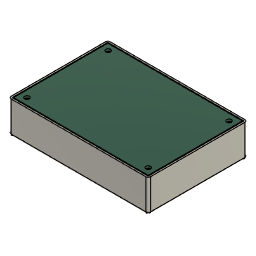
Commodore_KB_Tester_Rev2 v2 (Autodesk Fusion 360 design; units mm, degrees)
Autodesk Fusion 360 part; units mm, degrees
sketch "Sketch1" plane through (0, 0, 0) normal (0, 0, 1) x (1, 0, 0) in component "PCB"
  line L0 (100, 0) -> (100, 70)
  circle A0 centre (52, 35) radius 3.1
  circle A1 centre (35, 27) radius 3.1
  circle A2 centre (35, 42) radius 3.1
  line L1 (0, 0) -> (100, 0)
  line L2 (0, 70) -> (0, 0)
  circle A3 centre (52, 41.4) radius 1.2
  circle A4 centre (28.6, 27) radius 1.2
  line L3 (100, 70) -> (0, 70)
  circle A5 centre (28.6, 42) radius 1.2
  line L4 (99.15, 22.18) -> (97.6, 22.18)
  line L5 (97.6, 22.18) -> (97.6, 15.02)
  line L6 (88.4, 15.02) -> (97.6, 15.02)
  line L7 (97.6, 15.02) -> (99.15, 15.02)
  line L8 (97.6, 22.18) -> (88.4, 22.18)
  line L9 (94.5, 22.84) -> (94.7, 22.64)
  line L10 (94.7, 22.64) -> (93.4, 22.64)
  line L11 (93.4, 22.84) -> (93.4, 22.44)
  line L12 (99.15, 15.02) -> (99.15, 22.18)
  line L13 (72.2313, 9.5251) -> (67.6275, 9.5251)
  line L14 (72.2313, 8.5725) -> (72.2313, 9.5251)
  circle A6 centre (5, 5) radius 3.1789
  line L15 (2.54, 60) -> (2.54, 59)
  line L16 (2.54, 49.4) -> (2.54, 47.2)
  line L17 (14.04, 42) -> (18.34, 42)
  arc A7 (18.34, 49) -> (19.04, 49.7) centre (18.34, 49.7) ccw
  line L18 (18.34, 45.5) -> (16.54, 45.5)
  line L19 (67.6276, 8.5725) -> (72.2313, 8.5725)
  arc A8 (19.04, 52.3) -> (18.34, 53) centre (18.34, 52.3) ccw
  line L20 (2.54, 52.6) -> (2.54, 49.4)
  circle A9 centre (95, 65) radius 1.7463
  line L21 (2.54, 54.8) -> (2.54, 52.6)
  circle A10 centre (5, 5) radius 1.7463
  line L22 (19.04, 49.7) -> (19.04, 52.3)
  arc A11 (18.34, 42) -> (19.04, 42.7) centre (18.34, 42.7) ccw
  line L23 (67.6275, 9.5251) -> (67.6276, 8.5725)
  circle A12 centre (95, 65) radius 3.1789
  line L24 (16.54, 33) -> (18.34, 33)
  line L25 (19.04, 42.7) -> (19.04, 44.8)
  line L26 (13.64, 43) -> (14.04, 43)
  line L27 (16.04, 58.1) -> (16.34, 58.1)
  line L28 (2.54, 43) -> (1.54, 43)
  line L29 (2.54, 49.4) -> (14.04, 49.4)
  line L30 (14.04, 49.4) -> (14.04, 46.6)
  arc A13 (19.04, 59.3) -> (18.34, 60) centre (18.34, 59.3) ccw
  line L31 (2.54, 23) -> (2.54, 22)
  arc A14 (19.04, 44.8) -> (18.34, 45.5) centre (18.34, 44.8) ccw
  line L32 (18.34, 25.5) -> (16.54, 25.5)
  line L33 (0.84, 61.6) -> (0.84, 60)
  line L34 (14.04, 59) -> (14.04, 56.6)
  circle A15 centre (95, 5) radius 1.7463
  line L35 (0.74, 40.4) -> (0.74, 42)
  arc A16 (18.34, 22) -> (19.04, 22.7) centre (18.34, 22.7) ccw
  line L36 (1.54, 43) -> (1.54, 40.4)
  line L37 (18.34, 56.5) -> (16.54, 56.5)
  line L38 (2.54, 43) -> (11.44, 43)
  line L39 (0.04, 61.6) -> (0.04, 42)
  line L40 (2.54, 44.8) -> (2.54, 43)
  line L41 (1.54, 59) -> (2.54, 59)
  arc A17 (19.04, 24.8) -> (18.34, 25.5) centre (18.34, 24.8) ccw
  line L42 (16.34, 58.9) -> (16.04, 58.9)
  line L43 (2.54, 52.6) -> (14.04, 52.6)
  line L44 (14.04, 55.4) -> (14.04, 52.6)
  line L45 (14.04, 45.4) -> (14.04, 43)
  line L46 (16.04, 58.9) -> (16.04, 58.1)
  line L47 (2.54, 42) -> (14.04, 42)
  line L48 (16.54, 53) -> (18.34, 53)
  line L49 (2.54, 40) -> (2.54, 39)
  line L50 (2.54, 32.6) -> (2.54, 29.4)
  circle A18 centre (4.99, 65.33) radius 1.7463
  line L51 (2.54, 29.4) -> (2.54, 27.2)
  line L52 (16.54, 56.5) -> (16.54, 53)
  line L53 (2.54, 39) -> (2.54, 37.2)
  line L54 (16.54, 49) -> (18.34, 49)
  arc A19 (19.04, 32.3) -> (18.34, 33) centre (18.34, 32.3) ccw
  line L55 (0.74, 42) -> (0.04, 42)
  line L56 (2.54, 59) -> (2.54, 57.2)
  line L57 (14.04, 43) -> (14.04, 42)
  line L58 (0.84, 60) -> (1.54, 60)
  line L59 (16.04, 43.9) -> (16.04, 43.1)
  line L60 (2.54, 24.8) -> (2.54, 23)
  line L61 (16.34, 43.9) -> (16.04, 43.9)
  line L62 (2.54, 43) -> (2.54, 42)
  line L63 (14.04, 60) -> (2.54, 60)
  line L64 (14.04, 52.6) -> (14.04, 49.4)
  line L65 (16.54, 49) -> (16.54, 45.5)
  line L66 (0.74, 40.4) -> (1.54, 40.4)
  circle A20 centre (4.99, 65.33) radius 3.1789
  line L67 (2.54, 34.8) -> (2.54, 32.6)
  line L68 (16.04, 43.1) -> (16.34, 43.1)
  circle A21 centre (95, 5) radius 3.1789
  line L69 (1.54, 60) -> (1.54, 59)
  arc A22 (18.34, 56.5) -> (19.04, 57.2) centre (18.34, 57.2) ccw
  line L70 (0.04, 61.6) -> (0.84, 61.6)
  line L71 (13.64, 59) -> (14.04, 59)
  line L72 (14.04, 40) -> (14.04, 39)
  arc A23 (19.04, 39.3) -> (18.34, 40) centre (18.34, 39.3) ccw
  line L73 (18.34, 60) -> (14.04, 60)
  line L74 (16.04, 23.9) -> (16.04, 23.1)
  line L75 (14.5, 16.5) -> (14, 16.5)
  line L76 (19.04, 22.7) -> (19.04, 24.8)
  line L77 (14.04, 35.4) -> (14.04, 32.6)
  line L78 (14.04, 22) -> (18.34, 22)
  line L79 (18.34, 40) -> (14.04, 40)
  line L80 (16.04, 38.9) -> (16.04, 38.1)
  line L81 (16.04, 23.1) -> (18.04, 23.1)
  line L82 (2.54, 23) -> (1.54, 23)
  line L83 (2.54, 29.4) -> (14.04, 29.4)
  line L84 (0.04, 41.6) -> (0.84, 41.6)
  line L85 (14, 19.5) -> (14, 19.2)
  line L86 (3.5, 19.2) -> (3.5, 19.5)
  line L87 (18.34, 36.5) -> (16.54, 36.5)
  line L88 (14.04, 40) -> (2.54, 40)
  line L89 (14.04, 29.4) -> (14.04, 26.6)
  line L90 (0.74, 20.4) -> (0.74, 22)
  line L91 (14.04, 39) -> (14.04, 36.6)
  line L92 (0.74, 22) -> (0.04, 22)
  line L93 (16.54, 29) -> (18.34, 29)
  line L94 (14.04, 32.6) -> (14.04, 29.4)
  line L95 (19.04, 29.7) -> (19.04, 32.3)
  line L96 (1.54, 39) -> (2.54, 39)
  line L97 (13.64, 23) -> (14.04, 23)
  line L98 (16.54, 29) -> (16.54, 25.5)
  line L99 (14.5, 16.5) -> (14.5, 19.5)
  line L100 (16.54, 36.5) -> (16.54, 33)
  line L101 (18.04, 23.9) -> (16.04, 23.9)
  line L102 (1.54, 23) -> (1.54, 20.4)
  line L103 (0.84, 40) -> (1.54, 40)
  line L104 (18.04, 38.9) -> (16.04, 38.9)
  line L105 (2.54, 23) -> (11.44, 23)
  line L106 (1.54, 40) -> (1.54, 39)
  line L107 (16.04, 38.1) -> (18.04, 38.1)
  line L108 (91.3, 57.912) -> (91.4232, 57.912)
  line L109 (0.74, 20.4) -> (1.54, 20.4)
  line L110 (18.04, 38.1) -> (18.04, 38.9)
  line L111 (18.04, 23.1) -> (18.04, 23.9)
  line L112 (14.5, 13.5) -> (14.5, 13.8)
  line L113 (14, 19.2) -> (14, 16.5)
  line L114 (11.5, 10.8) -> (14, 10.8)
  line L115 (91.3, 58) -> (91.3, 57)
  line L116 (2.54, 59) -> (11.44, 59)
  line L117 (13.64, 39) -> (14.04, 39)
  line L118 (3.5, 10.8) -> (9.7, 10.8)
  arc A24 (18.34, 29) -> (19.04, 29.7) centre (18.34, 29.7) ccw
  line L119 (14.04, 23) -> (14.04, 22)
  arc A25 (18.34, 36.5) -> (19.04, 37.2) centre (18.34, 37.2) ccw
  line L120 (0.84, 41.6) -> (0.84, 40)
  line L121 (19.04, 39.3) -> (19.04, 37.2)
  line L122 (2.54, 22) -> (14.04, 22)
  line L123 (0.04, 41.6) -> (0.04, 22)
  line L124 (2.54, 32.6) -> (14.04, 32.6)
  line L125 (99.15, 43.96) -> (99.15, 59.04)
  line L126 (14.04, 60) -> (14.04, 59)
  line L127 (97.6, 59.04) -> (88.4, 59.04)
  line L128 (14.04, 25.4) -> (14.04, 23)
  line L129 (2.54, 39) -> (11.44, 39)
  line L130 (91.3, 21.14) -> (91.3, 20.14)
  line L131 (3.5, 10.8) -> (3.5, 19.2)
  line L132 (88.4, 22.18) -> (88.4, 15.02)
  line L133 (14.5, 10.5) -> (14, 10.5)
  line L134 (97.6, 29.44) -> (99.15, 29.44)
  line L135 (91.3, 57.15) -> (91.51, 57.15)
  line L136 (91.3, 57.785) -> (91.601, 57.785)
  line L137 (91.3, 57.531) -> (91.9566, 57.531)
  line L138 (97.6, 40.56) -> (88.4, 40.56)
  line L139 (97.6, 59.04) -> (97.6, 43.96)
  line L140 (92, 57.5) -> (91.3, 58)
  line L141 (91.3, 57.658) -> (91.7788, 57.658)
  line L142 (91.3, 39.37) -> (91.51, 39.37)
  line L143 (88.4, 29.44) -> (97.6, 29.44)
  line L144 (14, 13.5) -> (14, 10.8)
  line L145 (92, 39.02) -> (91.3, 39.52)
  line L146 (91.3, 39.243) -> (91.6878, 39.243)
  line L147 (3.5, 10.5) -> (3.5, 10.8)
  line L148 (99.15, 29.44) -> (99.15, 40.56)
  line L149 (91.3, 39.52) -> (91.3, 38.52)
  line L150 (91.3, 21.082) -> (91.3812, 21.082)
  line L151 (88.4, 59.04) -> (88.4, 43.96)
  line L152 (14, 13.5) -> (14.5, 13.5)
  line L153 (14.5, 13.5) -> (14.5, 10.5)
  line L154 (91.3, 57) -> (92, 57.5)
  line L155 (91.3, 57.023) -> (91.3322, 57.023)
  line L156 (91.3, 20.955) -> (91.559, 20.955)
  line L157 (94.7, 41.02) -> (93.4, 41.02)
  line L158 (14.5, 19.5) -> (14, 19.5)
  line L159 (14, 13.8) -> (14, 13.5)
  line L160 (14, 10.8) -> (14, 10.5)
  line L161 (91.3, 38.52) -> (92, 39.02)
  line L162 (0, 10.5) -> (3.5, 10.5)
  line L163 (94.5, 59.7) -> (94.7, 59.5)
  line L164 (93.4, 59.7) -> (93.4, 59.3)
  line L165 (88.4, 43.96) -> (97.6, 43.96)
  line L166 (97.6, 43.96) -> (99.15, 43.96)
  line L167 (91.3, 57.277) -> (91.6878, 57.277)
  line L168 (91.3, 57.404) -> (91.8656, 57.404)
  line L169 (14, 16.5) -> (14, 16.2)
  line L170 (91.3, 39.116) -> (91.8656, 39.116)
  line L171 (3.5, 19.5) -> (0, 19.5)
  line L172 (91.3, 20.447) -> (91.7298, 20.447)
  line L173 (91.3, 20.574) -> (91.9076, 20.574)
  line L174 (9.5, 10.5) -> (3.5, 10.5)
  line L175 (3.5, 19.5) -> (14, 19.5)
  line L176 (3.5, 19.2) -> (14, 19.2)
  line L177 (91.3, 20.193) -> (91.3742, 20.193)
  line L178 (14.5, 16.5) -> (14.5, 16.2)
  line L179 (91.3, 20.32) -> (91.552, 20.32)
  line L180 (91.3, 20.701) -> (91.9146, 20.701)
  line L181 (0, 19.5) -> (0, 10.5)
  line L182 (91.3, 20.828) -> (91.7368, 20.828)
  line L183 (91.3, 39.497) -> (91.3322, 39.497)
  line L184 (99.15, 59.04) -> (97.6, 59.04)
  line L185 (88.4, 40.56) -> (88.4, 29.44)
  line L186 (91.3, 20.14) -> (92, 20.64)
  line L187 (99.15, 40.56) -> (97.6, 40.56)
  line L188 (14, 10.5) -> (11.7, 10.5)
  line L189 (94.7, 59.5) -> (93.4, 59.5)
  line L190 (91.3, 38.862) -> (91.7788, 38.862)
  line L191 (91.3, 38.989) -> (91.9566, 38.989)
  line L192 (94.5, 41.22) -> (94.7, 41.02)
  arc A26 (38.7, 28.1) -> (38.7, 25.85) centre (34.9998, 26.975) ccw
  line L193 (37.25, 30.85) -> (32.75, 30.85)
  line L194 (92, 20.64) -> (91.3, 21.14)
  circle A27 centre (52, 35) radius 5.4
  line L195 (37.25, 30.85) -> (39.45, 27)
  circle A28 centre (35, 42) radius 5.4
  arc A29 (37.7, 25.5) -> (37.7, 28.5) centre (37.7, 27) ccw
  line L196 (39.45, 27) -> (37.25, 23.15)
  line L197 (93.4, 41.22) -> (93.4, 40.82)
  line L198 (91.3, 38.735) -> (91.601, 38.735)
  line L199 (91.3, 38.608) -> (91.4232, 38.608)
  line L200 (37.25, 45.85) -> (39.45, 42)
  line L201 (30.55, 42) -> (32.75, 38.15)
  line L202 (32.75, 45.85) -> (30.55, 42)
  line L203 (32.75, 30.85) -> (30.55, 27)
  line L204 (39.45, 42) -> (37.25, 38.15)
  line L205 (37.25, 23.15) -> (32.75, 23.15)
  circle A30 centre (35, 27) radius 5.4
  line L206 (55.85, 32.75) -> (52, 30.55)
  line L207 (52, 30.55) -> (48.15, 32.75)
  line L208 (30.55, 27) -> (32.75, 23.15)
  line L209 (37.25, 38.15) -> (32.75, 38.15)
  line L210 (55.85, 32.75) -> (55.85, 37.25)
  arc A31 (53.1, 31.3) -> (50.85, 31.3) centre (51.975, 35.0002) ccw
  arc A32 (38.7, 43.1) -> (38.7, 40.85) centre (34.9998, 41.975) ccw
  line L211 (37.25, 45.85) -> (32.75, 45.85)
  line L212 (48.15, 32.75) -> (48.15, 37.25)
  line L213 (52, 39.45) -> (48.15, 37.25)
  line L214 (55.85, 37.25) -> (52, 39.45)
  line L215 (97.6, 40.56) -> (97.6, 29.44)
  arc A33 (37.7, 40.5) -> (37.7, 43.5) centre (37.7, 42) ccw
  arc A34 (50.5, 32.3) -> (53.5, 32.3) centre (52, 32.3) ccw
  line L216 (93.4, 21.18) -> (93.4, 19.98)
  line L217 (94.6, 17.22) -> (93.4, 17.22)
  line L218 (93.4, 16.02) -> (94.6, 16.02)
  line L219 (93.4, 19.98) -> (94.6, 19.98)
  line L220 (94.6, 21.18) -> (93.4, 21.18)
  line L221 (93.4, 17.22) -> (93.4, 16.02)
  line L222 (18.04, 58.1) -> (18.04, 58.9)
  circle A35 centre (43, 9) radius 2
  line L223 (2.54, 57.2) -> (2.54, 54.8)
  circle A36 centre (62.05, 9) radius 5
  circle A37 centre (43, 61) radius 5
  line L224 (2.54, 37.2) -> (2.54, 34.8)
  line L225 (18.04, 58.9) -> (16.34, 58.9)
  circle A38 centre (62.05, 9) radius 2
  line L226 (93.4, 58.04) -> (93.4, 56.84)
  line L227 (14.04, 46.6) -> (14.04, 45.4)
  line L228 (94.6, 16.02) -> (94.6, 17.22)
  line L229 (18.04, 43.1) -> (18.04, 43.9)
  line L230 (16.34, 43.1) -> (18.04, 43.1)
  line L231 (94.6, 19.98) -> (94.6, 21.18)
  line L232 (11.44, 43) -> (13.64, 43)
  line L233 (14.04, 56.6) -> (14.04, 55.4)
  circle A39 centre (43, 9) radius 5
  line L234 (2.54, 47.2) -> (2.54, 44.8)
  circle A40 centre (78, 61) radius 2
  line L235 (14.04, 26.6) -> (14.04, 25.4)
  circle A41 centre (78, 9) radius 2
  line L236 (2.54, 27.2) -> (2.54, 24.8)
  circle A42 centre (78, 61) radius 5
  circle A43 centre (62.05, 61) radius 2
  circle A44 centre (78, 41.95) radius 2
  circle A45 centre (78, 28.05) radius 2
  circle A46 centre (78, 41.95) radius 5
  line L237 (11.44, 23) -> (13.64, 23)
  circle A47 centre (62.05, 61) radius 5
  line L238 (14.04, 36.6) -> (14.04, 35.4)
  line L239 (14, 16.2) -> (14, 13.8)
  line L240 (18.04, 43.9) -> (16.34, 43.9)
  line L241 (11.44, 39) -> (13.64, 39)
  circle A48 centre (43, 61) radius 2
  line L242 (16.34, 58.1) -> (18.04, 58.1)
  line L243 (10, 10.5) -> (11.2, 10.5)
  line L244 (11.44, 59) -> (13.64, 59)
  line L245 (11.2, 10) -> (10, 10)
  circle A49 centre (78, 9) radius 5
  line L246 (93.4, 56.84) -> (94.6, 56.84)
  line L247 (14.5, 13.8) -> (14.5, 16.2)
  line L248 (94.6, 35.6) -> (93.4, 35.6)
  line L249 (36.45, 28.5) -> (37.5, 28.5)
  line L250 (94.6, 31.64) -> (93.4, 31.64)
  line L251 (36.45, 43.5) -> (37.5, 43.5)
  line L252 (53.5, 35) -> (53.5, 33.55)
  line L253 (94.6, 46.16) -> (93.4, 46.16)
  line L254 (94.6, 39.56) -> (93.4, 39.56)
  line L255 (94.6, 56.84) -> (94.6, 58.04)
  line L256 (93.4, 52.88) -> (94.6, 52.88)
  line L257 (10, 10) -> (10, 10.5)
  line L258 (9.7, 10.8) -> (11.5, 10.8)
  line L259 (94.6, 38.36) -> (94.6, 39.56)
  line L260 (93.4, 48.92) -> (94.6, 48.92)
  line L261 (94.6, 48.92) -> (94.6, 50.12)
  arc A50 (53.5, 32.5) -> (50.5, 32.5) centre (52, 35) ccw
  line L262 (36.45, 40.5) -> (37.5, 40.5)
  line L263 (94.6, 54.08) -> (93.4, 54.08)
  arc A51 (36.45, 43.5) -> (36.45, 40.5) centre (35, 42) ccw
  arc A52 (37.5, 43.5) -> (37.5, 40.5) centre (35, 42) ccw
  line L264 (37.5, 28.5) -> (37.7, 28.5)
  line L265 (93.4, 31.64) -> (93.4, 30.44)
  line L266 (35, 25.5) -> (36.45, 25.5)
  line L267 (94.6, 34.4) -> (94.6, 35.6)
  line L268 (93.4, 46.16) -> (93.4, 44.96)
  line L269 (94.6, 44.96) -> (94.6, 46.16)
  line L270 (93.4, 30.44) -> (94.6, 30.44)
  line L271 (93.4, 50.12) -> (93.4, 48.92)
  line L272 (11.2, 10.5) -> (11.7, 10.5)
  line L273 (93.4, 34.4) -> (94.6, 34.4)
  line L274 (93.4, 35.6) -> (93.4, 34.4)
  line L275 (50.5, 35) -> (50.5, 33.55)
  line L276 (94.6, 52.88) -> (94.6, 54.08)
  line L277 (50.5, 32.5) -> (50.5, 32.3)
  line L278 (36.45, 25.5) -> (37.5, 25.5)
  line L279 (37.5, 25.5) -> (37.7, 25.5)
  line L280 (35, 28.5) -> (36.45, 28.5)
  circle A53 centre (78, 28.05) radius 5
  line L281 (9.5, 10.5) -> (10, 10.5)
  line L282 (11.2, 10.5) -> (11.2, 10)
  line L283 (37.5, 40.5) -> (37.7, 40.5)
  line L284 (93.4, 54.08) -> (93.4, 52.88)
  line L285 (94.6, 50.12) -> (93.4, 50.12)
  line L286 (53.5, 33.55) -> (53.5, 32.5)
  line L287 (93.4, 44.96) -> (94.6, 44.96)
  line L288 (94.6, 30.44) -> (94.6, 31.64)
  line L289 (94.6, 58.04) -> (93.4, 58.04)
  line L290 (35, 43.5) -> (36.45, 43.5)
  arc A54 (53.5, 35) -> (50.5, 35) centre (52, 35) ccw
  arc A55 (53.5, 33.55) -> (50.5, 33.55) centre (52, 35) ccw
  line L291 (35, 40.5) -> (36.45, 40.5)
  line L292 (93.4, 39.56) -> (93.4, 38.36)
  arc A56 (37.5, 28.5) -> (37.5, 25.5) centre (35, 27) ccw
  line L293 (93.4, 38.36) -> (94.6, 38.36)
  arc A57 (36.45, 28.5) -> (36.45, 25.5) centre (35, 27) ccw
  line L294 (53.5, 32.5) -> (53.5, 32.3)
  arc A58 (35, 28.5) -> (35, 25.5) centre (35, 27) ccw
  arc A59 (35, 43.5) -> (35, 40.5) centre (35, 42) ccw
  line L295 (37.5, 43.5) -> (37.7, 43.5)
  line L296 (50.5, 33.55) -> (50.5, 32.5)
  line L297 (-50, -35) -> (50, -35) construction
  line L298 (50, -35) -> (50, 35) construction
  line L299 (50, 35) -> (-50, 35) construction
  line L300 (-50, 35) -> (-50, -35) construction
  circle A60 centre (-45.01, 30.33) radius 1.7463 construction
  circle A61 centre (45, 30) radius 1.7463 construction
  circle A62 centre (45, -30) radius 1.7463 construction
  circle A63 centre (-45, -30) radius 1.7463 construction
extrude "Extrude1" add sketch "Sketch1" along normal blind 1.6 contours L0 L1 L2 L3 L99 L112 L133 L153 L158 L162 L171 L174 L175 L178 L188 L245 L247 L257 L272 L281 L282 | L2 L86 L131 L147 L162 L171 L181 | L114 L118 L147 L160 L174 L188 L243 L258 L272 L281 | L85 L86 L175 L176 | L113 L114 L118 L131 L144 L159 L169 L176 L239 L258 | L75 L85 L99 L113 L158 | L243 L245 L257 L282 | L75 L112 L152 L159 L169 L178 L239 L247 | L133 L144 L152 L153 L160 | A0 A34 A50 L277 L294 | A0 A34 L252 L275 L277 L286 A54 L294 L296 | A0 A34 | A50 L286 A55 L296 | L252 L275 A54 A55 | A1 A29 L249 L264 L266 L278 L279 L280 A58 | A1 A29 | A1 A29 L264 L279 A56 | L249 L278 A56 A57 | L266 L280 A57 A58 | A2 A33 L251 L262 L283 L290 L291 A59 L295 | A2 A33 | A2 A33 A52 L283 L295 | L251 L262 A51 A52 | A51 L290 L291 A59 | A3 A27 | A3 A27 | A3 A27 | A4 A30 | A4 A30 | A4 A30 | A5 A28 | A5 A28 | A5 A28 | L4 L5 L7 L12 | L5 L6 L8 L132 | L13 L14 L19 L23 | A6 | L15 L63 L71 L116 L126 L244 | L16 L20 L21 L28 L33 L35 L36 L39 L40 L41 L55 L56 L58 L66 L69 L70 L84 L120 L223 L234 | L21 L34 L43 L44 L56 L71 L116 L223 L233 L244 | L20 L29 L43 L64 | L16 L26 L29 L30 L38 L40 L45 L227 L232 L234 | L26 L38 L47 L57 L62 L232 | L35 L66 L84 L120 | L35 L50 L51 L53 L60 L66 L67 L82 L84 L90 L92 L96 L102 L103 L106 L109 L120 L123 L224 L236 | L53 L67 L77 L91 L117 L124 L129 L224 L238 L241 | L49 L72 L88 L117 L129 L241 | L31 L97 L105 L119 L122 L237 | L51 L60 L83 L89 L97 L105 L128 L235 L236 L237 | L24 L32 A16 A17 A19 L72 A23 L76 L77 L78 L79 L87 L89 L91 L93 L94 L95 L98 L100 A24 L119 A25 L121 L128 L235 L238 | L50 L83 L94 L124 | A12 | L27 L42 L46 L222 L225 L242 | L59 L61 L68 L229 L230 L240 | A20 | A21 | L74 L81 L101 L111 | L80 L104 L107 L110 | L108 L115 L140 | L108 L115 L136 L140 | L115 L136 L140 L141 | L115 L137 L140 L141 | L115 L137 L140 L154 L168 | L115 L154 L167 L168 | L115 L135 L154 L167 | L115 L135 L154 L155 | L115 L154 L155 | L125 L139 L166 L184 | L127 L139 L151 L165 | L130 L150 L194 | L130 L150 L156 L194 | L130 L156 L182 L194 | L130 L180 L182 L194 | L130 L173 L180 L186 L194 | L130 L172 L173 L186 | L130 L172 L179 L186 | L130 L177 L179 L186 | L130 L177 L186 | L134 L148 L187 L215 | L138 L143 L185 L215 | L142 L145 L149 L183 | L142 L145 L146 L149 | L145 L149 L183 | L145 L146 L149 L170 | L145 L149 L161 L170 L191 | L149 L161 L190 L191 | L149 L161 L190 L198 | L149 L161 L198 L199 | L149 L161 L199 | A26 L208 | A26 L193 L195 L196 L203 L205 L208 | A26 L205 L208 | A26 L205 | A26 L196 L205 | A26 L196 | L200 L201 L202 L204 L209 A32 L211 | L204 A32 | L204 L209 A32 | L201 A32 | L209 A32 | L201 L209 A32 | L206 L207 L210 A31 L212 L213 L214 | L207 A31 | L207 A31 L212 | A31 L213 | A31 L212 | A31 L212 L213 | L216 L219 L220 L231 | L217 L218 L221 L228 | A35 | A36 | A37 | A38 | L226 L246 L255 L289 | A39 | A40 | A41 | A42 | A43 | A44 | A45 | A46 | A47 | A48 | A49 | L248 L267 L273 L274 | L250 L265 L270 L288 | L253 L268 L269 L287 | L254 L259 L292 L293 | L256 L263 L276 L284 | L260 L261 L271 L285 | A53 makes body 1 in component "PCB"
ref_plane "WorkPlane1" through (50, 35, -21) normal (0, 0, 1) x (1, 0, 0) in component "KB_Tester_bottom_shell_Rev2"
sketch "Sketch1 (2)" plane through (50, 35, -21) normal (0, 0, 1) x (1, 0, 0) in component "KB_Tester_bottom_shell_Rev2"
  line L0 (-50, -35) -> (50, -35) construction
  line L1 (50, -35) -> (50, 35) construction
  line L2 (50, 35) -> (-50, 35) construction
  line L3 (-50, 35) -> (-50, -35) construction
  circle A0 centre (-45.01, 30.33) radius 1.7463 construction
  circle A1 centre (45, 30) radius 1.7463 construction
  circle A2 centre (45, -30) radius 1.7463 construction
  circle A3 centre (-45, -30) radius 1.7463 construction
  line L4 (50, -35.5) -> (-50, -35.5)
  line L5 (-50.5, -35) -> (-50.5, 35)
  line L6 (-50, 35.5) -> (50, 35.5)
  line L7 (50.5, 35) -> (50.5, -35)
  arc A4 (50.5, 35) -> (50, 35.5) centre (50, 35) ccw
  arc A5 (-50, 35.5) -> (-50.5, 35) centre (-50, 35) ccw
  arc A6 (-50.5, -35) -> (-50, -35.5) centre (-50, -35) ccw
  arc A7 (50, -35.5) -> (50.5, -35) centre (50, -35) ccw
  line L8 (-47, 34) -> (47, 34)
  line L9 (-49, -32) -> (-49, 32)
  line L10 (47, -34) -> (-47, -34)
  line L11 (49, 32) -> (49, -32)
  arc A8 (51.75, 35) -> (50, 36.75) centre (50, 35) ccw
  line L12 (-50, 36.75) -> (50, 36.75)
  arc A9 (-50, 36.75) -> (-51.75, 35) centre (-50, 35) ccw
  line L13 (-51.75, -35) -> (-51.75, 35)
  arc A10 (-51.75, -35) -> (-50, -36.75) centre (-50, -35) ccw
  line L14 (50, -36.75) -> (-50, -36.75)
  arc A11 (50, -36.75) -> (51.75, -35) centre (50, -35) ccw
  line L15 (51.75, 35) -> (51.75, -35)
  arc A12 (47, -34) -> (49, -32) centre (47, -32) ccw
  arc A13 (-49, -32) -> (-47, -34) centre (-47, -32) ccw
  arc A14 (-47, 34) -> (-49, 32) centre (-47, 32) ccw
  arc A15 (49, 32) -> (47, 34) centre (47, 32) ccw
  circle A16 centre (45, -30) radius 1.25
  circle A17 centre (-45, -30) radius 1.25
  circle A18 centre (-45.01, 30.33) radius 1.25
  circle A19 centre (45, 30) radius 1.25
  line L16 (49, 26) -> (45, 26)
  line L17 (41, 34) -> (41, 30)
  arc A20 (41, 30) -> (45, 26) centre (45, 30) ccw
  line L18 (0, 0) -> (-60, 0) construction
  line L19 (0, 0) -> (0, 45) construction
  line L20 (-49, 26) -> (-45, 26)
  arc A21 (-45, 26) -> (-41, 30) centre (-45, 30) ccw
  line L21 (-41, 34) -> (-41, 30)
  line L22 (49, -26) -> (45, -26)
  arc A22 (45, -26) -> (41, -30) centre (45, -30) ccw
  line L23 (41, -34) -> (41, -30)
  line L24 (-49, -26) -> (-45, -26)
  arc A23 (-41, -30) -> (-45, -26) centre (-45, -30) ccw
  line L25 (-41, -34) -> (-41, -30)
  dimension "d9" = 0.5
  dimension "d10" = 0.5
  dimension "d11" = 0.5
  dimension "d12" = 0.5
  dimension "d13" = 0.5
  dimension "d15" = -1.25
  dimension "d16" = 2
  dimension "d18" = 2.5
  dimension "d19" = 2.5
  dimension "d20" = 2.5
  dimension "d21" = 2.5
  dimension "d23" = 4
  constraint horizontal L4
  constraint vertical L5
  constraint horizontal L6
  constraint vertical L7
  constraint tangent L6 A4
  constraint tangent L7 A4
  constraint tangent L5 A5
  constraint tangent L6 A5
  constraint equal A4 A5
  constraint tangent L4 A6
  constraint tangent L5 A6
  constraint equal A4 A6
  constraint tangent L4 A7
  constraint tangent L7 A7
  constraint equal A4 A7
  constraint tangent L10 A12
  constraint tangent L11 A12
  constraint tangent L9 A13
  constraint tangent L10 A13
  constraint equal A12 A13
  constraint tangent L8 A14
  constraint tangent L9 A14
  constraint equal A12 A14
  constraint tangent L8 A15
  constraint tangent L11 A15
  constraint equal A12 A15
  constraint concentric A2 A16
  constraint concentric A3 A17
  constraint concentric A0 A18
  constraint concentric A1 A19
  constraint concentric A19 A20
  constraint coincident L11 L16.start
  constraint perpendicular L11 L16
  constraint tangent L16 A20
  constraint coincident L8 L17.start
  constraint perpendicular L8 L17
  constraint tangent L17 A20
  constraint coincident L18.start L19.start
  constraint perpendicular L13 L18
  constraint perpendicular L12 L19
  constraint symmetric L16.start L19 L20.start
  constraint symmetric L16.end L19 L20.end
  constraint symmetric L17.start L19 L21.start
  constraint symmetric L17.end L19 A21.end
  constraint symmetric A20 L19 A21
  constraint symmetric L16.start L18 L22.start
  constraint symmetric L16.end L18 L22.end
  constraint symmetric L17.start L18 L23.start
  constraint symmetric L17.end L18 A22.end
  constraint symmetric A20 L18 A22
  constraint symmetric L19 L22.start L24.start
  constraint symmetric L19 L22.end L24.end
  constraint symmetric L19 A22.end A23.start
  constraint symmetric L19 A22 A23
  constraint symmetric L19 L23.start L25.start
  measures "d9" distance of L0 L4
  measures "d10" distance of L2 L6
  measures "d11" distance of L1 L7
  measures "d12" distance of L3 L5
  measures "d13" radius of A4
  measures "d16" radius of A12
  measures "d18" diameter of A16
  measures "d19" diameter of A17
  measures "d20" diameter of A18
  measures "d21" diameter of A19
  measures "d23" radius of A20
extrude "Extrude1'" add sketch "Sketch1 (2)" along normal blind 21 separate body contours L4 L5 L6 L7 A4 A5 A6 A7 | L8 L9 A14 L20 A21 L21 | L8 L11 A15 L16 L17 A20 | L9 L10 A13 L24 A23 L25 | L10 L11 A12 L22 A22 L23 makes body 2 in component "KB_Tester_bottom_shell_Rev2"
extrude "Extrude2" add sketch "Sketch1 (2)" along normal blind 22.6 contours A8 L12 A9 L13 A10 L14 A11 L15 bodies 2 in component "KB_Tester_bottom_shell_Rev2"
extrude "Extrude3" add sketch "Sketch1 (2)" against normal blind 1.5 contours L4 L5 L6 L7 A4 A5 A6 A7 | L8 L9 A14 L20 A21 L21 | L8 L9 L10 L11 L16 L17 A20 L20 A21 L21 L22 A22 L23 L24 A23 L25 | L8 L11 A15 L16 L17 A20 | L9 L10 A13 L24 A23 L25 | L10 L11 A12 L22 A22 L23 | A8 L12 A9 L13 A10 L14 A11 L15 | A16 | A17 | A18 | A19 bodies 2 in component "KB_Tester_bottom_shell_Rev2"
fillet "Fillet1" radius 1 8 edges at (91, 1, -10.5) (99, 9, -10.5) (99, 61, -10.5) (91, 69, -10.5) (9, 69, -10.5) (1, 61, -10.5) (1, 9, -10.5) (9, 1, -10.5) on bodies 2 in component "KB_Tester_bottom_shell_Rev2"
fillet "Fillet2" radius 1 24 edges at (9.2929, 1.2929, -21) (9, 3.5, -21) (7.8284, 7.8284, -21) (3.5, 9, -21) (1.2929, 9.2929, -21) (1, 35, -21) (1.2929, 60.7071, -21) (3.5, 61, -21) (7.8284, 62.1716, -21) (9, 66.5, -21) (9.2929, 68.7071, -21) (50, 69, -21) (90.7071, 68.7071, -21) (91, 66.5, -21) (92.1716, 62.1716, -21) (96.5, 61, -21) (98.7071, 60.7071, -21) (99, 35, -21) (98.7071, 9.2929, -21) (96.5, 9, -21) (92.1716, 7.8284, -21) (91, 3.5, -21) (90.7071, 1.2929, -21) (50, 1, -21) on bodies 2 in component "KB_Tester_bottom_shell_Rev2"
fillet "Fillet3" radius 1.5 8 edges at (101.75, 35, -22.5) (101.2374, -1.2374, -22.5) (50, -1.75, -22.5) (-1.2374, -1.2374, -22.5) (-1.75, 35, -22.5) (-1.2374, 71.2374, -22.5) (50, 71.75, -22.5) (101.2374, 71.2374, -22.5) on bodies 2 in component "KB_Tester_bottom_shell_Rev2"
component "PCB" placed x (1, 0, 0) y (0, 1, 0) z (0, 0, 1) at (0, 0, 0)
component "KB_Tester_bottom_shell_Rev2" placed x (1, 0, 0) y (0, 1, 0) z (0, 0, 1) at (0, 0, 0)
equation "pcb = 1.6 mm"
equation "d2 = pcb"
equation "below = 21 mm"
equation "bottom = 1.5 mm"
equation "side = 2.5 mm"
equation "d7 = -below - pcb"
equation "dist = 0.5 mm"
equation "d9 = dist"
equation "d10 = dist"
equation "d11 = dist"
equation "d12 = dist"
equation "d13 = dist"
equation "d15 = -side / 2"
equation "drill = 2.5 mm"
equation "d18 = drill"
equation "d19 = drill"
equation "d20 = drill"
equation "d21 = drill"
equation "postradius = 1.5 mm + drill"
equation "d23 = postradius"
equation "d24 = below"
equation "d26 = below + pcb"
equation "d28 = -bottom"
equation "d35 = bottom"
